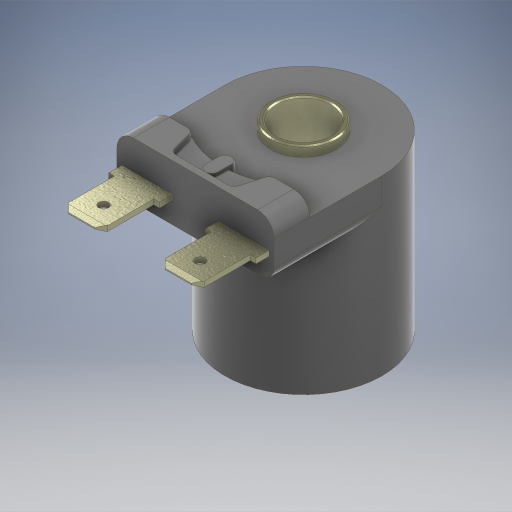
# Autodesk Inventor part: Solenoid
Saved by Autodesk Inventor 2024.1 (Build 281209000, 209)
## iProperties
Created: 2023-11-09
Part Number: Solenoid
Material: Steel, Galvanized
Document SubType Name: Modeling
Designer: Glen Collingwood
Density: 7.85 g/cm^3
Appearance: Galvanized
Author: Glen Collingwood
Autodesk Inventor part; units mm, degrees
sketch "Sketch1" plane through (0, 0, 0) normal (0, 1, 0) x (-1, 0, 0)
  circle A0 centre (0, 0) radius 5
  circle A1 centre (0, 0) radius 4.2
  dimension "d0" = 10
  dimension "d1" = 8.4
  constraints: 2 centre point, 2 coincident
  measures "d0" diameter of A0
  measures "d1" diameter of A1
extrude "Extrusion1" add sketch "Sketch1" along normal blind 30
ref_plane "Work Plane1" through (0, 2, 0) normal (0, -1, 0) x (1, 0, 0)
sketch "Sketch2" plane through (0, 2, 0) normal (0, -1, 0) x (1, 0, 0)
  circle A0 centre (0, 0) radius 4.2 projected
  circle A1 centre (0, 0) radius 5 projected
  circle A2 centre (0, 0) radius 12
  dimension "d5" = 24
  constraints: 1 centre point, 1 coincident
  measures "d5" diameter of A2
extrude "Extrusion2" add sketch "Sketch2" against normal blind 26.5 separate body contours A2
ref_plane "Work Plane2" through (0, 2, 12) normal (0, 0, 1) x (1, 0, 0)
sketch "Sketch3" plane through (0, 2, 12) normal (0, 0, 1) x (1, 0, 0)
  line L0 (-12, 29) -> (12, 29)
  line L1 (12, 29) -> (12, 20.5)
  line L2 (12, 20.5) -> (-12, 20.5)
  line L3 (-12, 20.5) -> (-12, 29)
  line L4 (5, 28) -> (-5, 28) projected
  line L5 (-12, 26.5) -> (12, 26.5)
  line L6 (12, 26.5) -> (-12, 26.5) projected
  point P0 (0, -2)
  point P1 (0, 20.5)
  dimension "d8" = 24
  dimension "d9" = 8.5
  dimension "d10" = 1
  constraints: 10 end point, 2 parallel, 2 perpendicular, 2 point on line, 1 collinear, 1 horizontal, 1 midpoint, 1 vertical alignment
  measures "d8" distance of L1.end L2.end
  measures "d9" distance of L0.end L1.end
  measures "d10" distance between parallel lines of L4 L0
extrude "Extrusion3" add sketch "Sketch3" against normal up to next contours L5 L1 L2 L3 bodies 2
sketch "Sketch4" plane through (0, 2, 12) normal (0, 0, 1) x (1, 0, 0)
  line L0 (-12, 0) -> (-12, 26.5) projected
  line L1 (-12, 20.5) -> (12, 20.5)
  line L2 (12, 20.5) -> (12, 29)
  line L3 (12, 29) -> (-12, 29)
  line L4 (-12, 29) -> (-12, 20.5)
  line L5 (12, 20.5) -> (12, 26.5) projected
  line L6 (0, 20.5) -> (12, 20.5) projected
  point P0 (0, -2)
  point P1 (-12, 26.5)
  dimension "d13" = 8.5
  constraints: 8 end point, 2 collinear, 2 parallel, 1 horizontal, 1 perpendicular, 1 point on line
  measures "d13" distance of L1.end L2.end
extrude "Extrusion4" add sketch "Sketch4" along normal blind 4.5 bodies 2
sketch "Sketch6" plane through (0, 2, 12) normal (0, 0, -1) x (-1, 0, 0)
  line L0 (12, 20.5) -> (0, 20.5) projected
  line L1 (0, 20.5) -> (-12, 20.5) projected
  line L2 (-12, 20.5) -> (-12, 26.5) projected
  line L3 (-12, 26.5) -> (-12, 29) projected
  line L4 (-12, 29) -> (12, 29) projected
  line L5 (12, 29) -> (12, 26.5) projected
  line L6 (12, 26.5) -> (12, 20.5) projected
  line L7 (0, 0) -> (0, 20.5) projected
  line L8 (12, 26.5) -> (-12, 26.5) projected
  point P0 (0, -2)
extrude "Extrusion5" add sketch "Sketch6" along normal blind 1 contours L8 L3 L4 L5 bodies 2
fillet "Fillet1" radius 2 2 edges at (12, 22.5, 8.25) (-12, 22.5, 8.25)
fillet "Fillet2" radius 2.5 2 edges at (-12, 31, 13.75) (12, 31, 13.75)
sketch "Sketch5" plane through (-9.5, 31, 12) normal (0, 1, 0) x (1, 0, 0)
  line L0 (19, 1) -> (19, -4.5) projected
  line L1 (19, -4.5) -> (0, -4.5) projected
  line L2 (0, -4.5) -> (0, 1) projected
  circle A0 centre (9.5, 12) radius 12.5
  line L3 (0, 1) -> (19, 1) projected
  dimension "d18" = 25
  constraints: 1 centre point, 1 coincident
  measures "d18" diameter of A0
extrude "Extrusion6" cut sketch "Sketch5" against normal up to surface (2.5 mm away) contours L3 A0 | A0 L3 bodies 2
sketch "Sketch7" plane through (-9.5, 31, 16.5) normal (0, 1, 0) x (1, 0, 0)
  line L0 (0, 5.5) -> (3.5628, 5.5) projected
  line L1 (1.2539, 5.5) -> (17.7461, 5.5)
  line L2 (17.7461, 5.5) -> (17.7461, 1)
  line L3 (17.7461, 1) -> (1.2539, 1)
  line L4 (1.2539, 1) -> (1.2539, 5.5)
  line L5 (19, 0) -> (0, 0) projected
  line L6 (15.4372, 5.5) -> (14.2314, 1)
  line L7 (3.5628, 5.5) -> (4.7686, 1)
  point P0 (9.5, 16.5)
  point P1 (9.5, 0)
  point P2 (9.5, 1)
  dimension "d23" = 1
  dimension "d24" = 105
  dimension "d25" = 105
  constraints: 12 end point, 3 point on line, 2 midpoint, 2 parallel, 1 horizontal, 1 perpendicular, 1 vertical alignment
  measures "d23" distance between parallel lines of L5 L3
  measures "d24" angle of L0 L7
  measures "d25" angle of L1 L6
extrude "Extrusion7" cut sketch "Sketch7" against normal blind 1 contours L1 L6 L3 L7 bodies 2
fillet "Fillet3" radius 1 4 edges at (5.9372, 30.5, 11) (-5.9372, 30.5, 11) (4.7314, 30.5, 15.5) (-4.7314, 30.5, 15.5)
sketch "Sketch8" plane through (0, 28.5, 0) normal (0, 1, 0) x (1, 0, 0)
  line L0 (0, -12) -> (0, -14) construction
  line L1 (1, -12) -> (1, -14)
  line L2 (-1, -14) -> (-1, -12)
  arc A0 (1, -12) -> (-1, -12) centre (0, -12) ccw
  arc A1 (-1, -14) -> (1, -14) centre (0, -14) ccw
  line L3 (9.5, -11) -> (9.5, -16.5) projected
  point P0 (0, 0)
  point P1 (0, -13)
  dimension "d29" = 2
  dimension "d30" = 12
  dimension "d31" = 2
  constraints: 8 end point, 4 point on circle, 4 tangent, 2 centre point, 2 parallel, 1 midpoint, 1 vertical
  measures "d29" distance between parallel lines of L1 L2
  measures "d30" distance of point (0, 0) L0.start
  measures "d31" distance of L0.start L0.end
extrude "Extrusion8" add sketch "Sketch8" along normal blind 2 bodies 2
chamfer "Chamfer1" distance 0.2 angle 45 2 edges at (4.2, 30, 0) (5, 30, 0)
ref_plane "Work Plane3" through (-9.5, 26.5, 16.5) normal (0, 1, 0) x (1, 0, 0)
sketch "Sketch9" plane through (-9.5, 26.5, 16.5) normal (0, 1, 0) x (1, 0, 0)
  line L0 (-1.75, 5) -> (6, 5)
  line L1 (6, 5) -> (6, -10)
  line L2 (6, -10) -> (-1.75, -10)
  line L3 (-1.75, -10) -> (-1.75, 5)
  line L4 (-0.5, 0) -> (19.5, 0) projected
  line L5 (-1.75, -10) -> (-0.875, -10)
  line L6 (-0.875, -10) -> (-0.875, -2)
  line L7 (-0.875, -2) -> (-1.75, -2)
  line L8 (-1.75, -2) -> (-1.75, -10)
  line L9 (6, -10) -> (5.125, -10)
  line L10 (5.125, -10) -> (5.125, -2)
  line L11 (5.125, -2) -> (6, -2)
  line L12 (6, -2) -> (6, -10)
  line L13 (-0.5, 0) -> (-2.5, 0) projected
  point P0 (9.5, 16.5)
  point P1 (9.5, 0)
  point P2 (2.125, -10)
  point P3 (-1.75, -2)
  point P4 (-0.875, -10)
  point P5 (5.125, -10)
  point P6 (6, -2)
  dimension "d38" = 7.75
  dimension "d40" = 11.25
  dimension "d41" = 10
  dimension "d42" = 5
  dimension "d43" = 6
  dimension "d44" = 3
  dimension "d45" = 2
  constraints: 24 end point, 6 parallel, 3 horizontal, 3 perpendicular, 2 midpoint, 1 point on line
  measures "d38" distance of L1.end L2.end
  measures "d40" distance from line of point (9.5, 0) L3
  measures "d41" distance from line of point (2.125, -10) L4
  measures "d42" distance between parallel lines of L4 L0
  measures "d43" distance between parallel lines of L10 L6
  measures "d44" distance from line of point (2.125, -10) L10
  measures "d45" distance between parallel lines of L13 L7
extrude "Extrusion9" add sketch "Sketch9" against normal blind 0.8 separate body contours L0 L1 L4 L13 L3 | L13 L4 L1 L11 L10 L2 L6 L7 L3
chamfer "Chamfer2" distance 1 angle 45 2 edges at (-4.375, 26.1, 26.5) (-10.375, 26.1, 26.5)
chamfer "Chamfer3" distance 0.8 distance2 0.3 1 edges at (-7.375, 26.5, 26.5) measured on face at (-7.375, 26.5, 26)
chamfer "Chamfer4" distance 0.8 distance2 0.3 1 edges at (-7.375, 25.7, 26.5) measured on face at (-7.375, 25.7, 26)
sketch "Sketch10" plane through (-9.5, 26.5, 16.5) normal (0, 1, 0) x (1, 0, 0)
  line L0 (0.125, -10) -> (4.125, -10) projected
  line L1 (2.125, -10) -> (2.125, -6.661)
  line L2 (2.125, -6.661) -> (2.125, -10.661)
  point P0 (9.5, 16.5)
  dimension "d57" = 4
  constraints: 4 end point, 1 midpoint, 1 perpendicular, 1 point on line
  measures "d57" distance of L1.end L2.end
hole "Hole1" at (-7.375, 26.5, 23.161) direction (0, -1, 0) diameter 1.5 end through all bodies 3
mirror "Mirror1" about plane through (0, 0, 0) normal (1, 0, 0) of "Extrusion9", "Chamfer2", "Chamfer3", "Chamfer4", "Hole1" bodies 3
equation "\"d25\" = d24"
equation "\"d44\" = 0.5 * d43"
body "Solid1"
body "Solid2"
body "Solid4"
